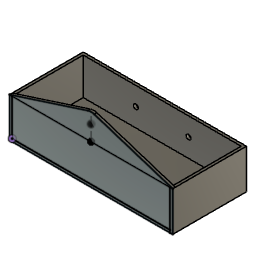
bagDispenser (Autodesk Fusion 360 design; units mm, degrees)
Autodesk Fusion 360 part; units mm, degrees
sketch "Esquisse1" plane through (0, 0, 0) normal (0, 1, 0) x (1, 0, 0)
  line L0 (0, 0) -> (150, 0)
  line L1 (150, 0) -> (150, -35)
  line L2 (150, -35) -> (0, -35)
  line L3 (0, -35) -> (0, 0)
  line L4 (75, -35) -> (75, -60) construction
  line L5 (0, 0) -> (150, 0)
  line L6 (150, 0) -> (150, 2.5)
  line L7 (150, 2.5) -> (0, 2.5)
  line L8 (0, 2.5) -> (0, 0)
  line L9 (150, -35) -> (152.5, -35)
  line L10 (152.5, -35) -> (152.5, 2.5)
  line L11 (152.5, 2.5) -> (150, 2.5)
  line L12 (150, 2.5) -> (150, -35)
  line L13 (0, -35) -> (-2.5, -35)
  line L14 (-2.5, -35) -> (-2.5, 2.5)
  line L15 (-2.5, 2.5) -> (0, 2.5)
  line L16 (0, 2.5) -> (0, -35)
  line L17 (-2.5, -35) -> (71.93, -59.0097)
  line L18 (78.07, -59.0097) -> (152.5, -35)
  arc A0 (71.93, -59.0097) -> (78.07, -59.0097) centre (75, -49.4926) ccw
  point P0 (75, -35)
  dimension "d6" = 150
  dimension "d7" = 35
  dimension "d8" = 25
  dimension "d13" = 150
  dimension "d14" = 2.5
  dimension "d15" = 2.5
  dimension "d16" = 37.5
  dimension "d17" = 2.5
  dimension "d18" = 37.5
  dimension "d19" = 10
  constraint horizontal L0
  constraint vertical L1
  constraint horizontal L2
  constraint vertical L3
  constraint coincident L0.start L3.end
  constraint coincident L2 P0
  constraint midpoint L2 P0
  constraint coincident P0 L4.start
  constraint perpendicular L2 L4
  constraint horizontal L5
  constraint vertical L6
  constraint horizontal L7
  constraint vertical L8
  constraint horizontal L9
  constraint vertical L10
  constraint horizontal L11
  constraint vertical L12
  constraint horizontal L13
  constraint vertical L14
  constraint horizontal L15
  constraint vertical L16
  constraint coincident L4.end L17
  constraint coincident L4.end L18
  constraint tangent L17 A0
  constraint tangent L18 A0
  measures "d6" distance of L0.start L0.end
  measures "d7" distance of L0.start L2.end
  measures "d8" distance of P0 L4.end
  measures "d13" distance of L0.start L0.end
  measures "d14" distance of L0.start L7.end
  measures "d15" distance of L1.end L9.end
  measures "d16" distance of L1.end L6.end
  measures "d17" distance of L2.end L13.end
  measures "d18" distance of L2.end L7.end
  measures "d19" radius of A0
extrude "Extrusion2" add sketch "Esquisse1" along normal blind 2.5 contours L0 L1 L2 L3 L5 L12 L16 | L2 L9 L13 L17 L18 A0
extrude "Extrusion3" add sketch "Esquisse1" along normal blind 70 contours L0 L5 L6 L7 L8 L12 L16 | L3 L8 L13 L14 L15 L16 | L1 L6 L9 L10 L11 L12
ref_plane "Plan de construction1" through (75, 70, 16.25) normal (0, 1, 0) x (0, 0, 1)
sketch "Esquisse2" plane through (75, 70, 16.25) normal (0, 1, 0) x (1, 0, 0)
  line L0 (-75, 16.25) -> (-75, -18.75)
  line L1 (-75, -18.75) -> (-77.5, -18.75)
  line L2 (-77.5, -18.75) -> (-3.07, -42.7597)
  arc A0 (-3.07, -42.7597) -> (3.07, -42.7597) centre (0, -33.2426) ccw
  line L3 (3.07, -42.7597) -> (77.5, -18.75)
  line L4 (77.5, -18.75) -> (75, -18.75)
  line L5 (75, -18.75) -> (75, 16.25)
  line L6 (75, 16.25) -> (-75, 16.25)
  line L7 (75, -18.75) -> (-75, -18.75)
  line L8 (-75, -18.75) -> (-75, 16.25)
  line L9 (-75, 16.25) -> (75, 16.25)
  line L10 (75, 16.25) -> (75, -18.75)
  line L11 (75, -1.25) -> (-75, -1.25) construction
  line L12 (75, -1.25) -> (25, -1.25) construction
  line L13 (-75, -1.25) -> (-25, -1.25) construction
  circle A1 centre (25, -1.25) radius 2.25
  circle A2 centre (-25, -1.25) radius 2.25
  point P0 (75, -1.25)
  point P1 (-75, -1.25)
  dimension "d27" = 50
  dimension "d28" = 50
  dimension "d30" = 4.5
  dimension "d31" = 4.5
  constraint horizontal L7
  constraint vertical L8
  constraint horizontal L9
  constraint vertical L10
  constraint coincident L0.start L6.end
  constraint coincident L4.end L5.start
  constraint coincident L10 P0
  constraint midpoint L10 P0
  constraint coincident L8 P1
  constraint midpoint L8 P1
  constraint coincident P0 L11.start
  constraint coincident P1 L11.end
  constraint perpendicular L5 L12
  constraint perpendicular L0 L13
  constraint coincident L12.end A1.centre
  constraint coincident L13.end A2.centre
  measures "d27" distance of P0 L12.end
  measures "d28" distance of P1 L13.end
  measures "d30" diameter of A1
  measures "d31" diameter of A2
extrude "Extrusion4" add sketch "Esquisse2" against normal blind 2.5 contours L0 L5 L6 L7 L8 L9 L10 | A1 | A2
extrude "Extrusion5" cut sketch "Esquisse2" against normal blind 2.5 contours A1 | A2
equation "bagWidth = 150 mm"
equation "bagThickness = 65 mm"
equation "dispenserBorderHeight = 35 mm"
equation "dispenserTriangleHeight = 25 mm"
equation "dispenserThickness = 2.5 mm"
equation "d6 = bagWidth"
equation "d7 = dispenserBorderHeight"
equation "d8 = dispenserTriangleHeight"
equation "dispenserTriangleRoundCorner = 10 mm"
equation "d13 = bagWidth"
equation "d14 = dispenserThickness"
equation "d15 = dispenserThickness"
equation "d16 = dispenserBorderHeight + dispenserThickness"
equation "d17 = dispenserThickness"
equation "d18 = dispenserBorderHeight + dispenserThickness"
equation "d19 = dispenserTriangleRoundCorner"
equation "d20 = dispenserThickness"
equation "d22 = ( 2 * dispenserThickness ) + bagThickness"
equation "d25 = -dispenserThickness"
equation "d27 = bagWidth / 3"
equation "d28 = bagWidth / 3"
equation "screwHoleDiameter = 4.5 mm"
equation "d30 = screwHoleDiameter"
equation "d31 = screwHoleDiameter"
equation "d32 = -dispenserThickness"
